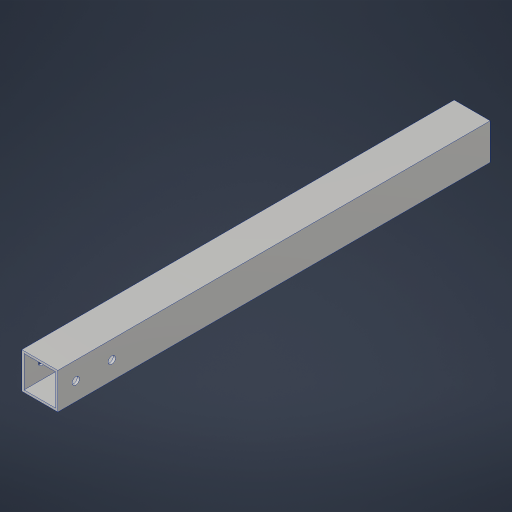
# Autodesk Inventor part: CL4-007
Saved by Autodesk Inventor 2023.4 (Build 274418000, 418)
## iProperties
RuleStatus: InUse
Created: 2025-02-03
Part Number: CL4-007
Material: Aluminum 6061
Document SubType Name: Modeling
Designer: brand
Mass: 304.185 g
Surface Area: 718.547 cm^2
Volume: 112.661 cm^3
Density: 2.7 g/cm^3
Appearance: Aluminum - Flat
AfterDocNew0: SHOW
AfterDocOpen0: SHOW
Author: brand
Autodesk Inventor part; units mm, degrees
ref_plane "YZ Plane" through (0, 0, 0) normal (1, 0, 0) x (0, 1, 0)
ref_plane "XZ Plane" through (0, 0, 0) normal (0, 1, 0) x (-1, 0, 0)
ref_plane "XY Plane" through (0, 0, 0) normal (0, 0, 1) x (1, 0, 0)
sketch "Sketch1" plane through (0, 0, 0) normal (0, 0, 1) x (1, 0, 0)
  line L0 (-12.7, -12.7) -> (12.7, -12.7)
  line L1 (12.7, -12.7) -> (12.7, 12.7)
  line L2 (12.7, 12.7) -> (-12.7, 12.7)
  line L3 (-12.7, 12.7) -> (-12.7, -12.7)
  line L4 (-12.7, -12.7) -> (12.7, 12.7) construction
  line L5 (12.7, -12.7) -> (-12.7, 12.7) construction
  line L6 (-11.1125, 11.1125) -> (11.1125, 11.1125)
  line L7 (11.1125, 11.1125) -> (11.1125, -11.1125)
  line L8 (11.1125, -11.1125) -> (-11.1125, -11.1125)
  line L9 (-11.1125, -11.1125) -> (-11.1125, 11.1125)
  point P0 (0, 0)
  dimension "width" = 25.4
  dimension "height" = 25.4
  dimension "thickness" = 1.5875
  constraints: 20 end point, 4 parallel, 2 midpoint, 2 perpendicular, 1 horizontal, 3 other
  measures "width" distance of L2.end L1.end
  measures "height" distance of L1.end L0.end
  measures "thickness" distance between parallel lines of L2 L6
extrude "Extrusion1" add sketch "Sketch1" along normal mid plane 304.8
sketch "Sketch2" plane through (12.7, -12.7, 152.4) normal (1, 0, 0) x (0, 0, -1)
  line L0 (304.8, 25.4) -> (304.8, 0) construction
  line L1 (304.8, 0) -> (0, 0) construction
  line L2 (0, 0) -> (0, 25.4) construction
  line L3 (0, 25.4) -> (304.8, 25.4) construction
  point P0 (152.4, 12.7)
  point P1 (12.7, 12.7)
  point P2 (38.1, 12.7)
  point P3 (0, 12.7)
  dimension "d5" = 25.4
  dimension "d6" = 12.7
  constraints: 2 horizontal alignment, 1 midpoint
  measures "d5" distance of point (38.1, 12.7) point (12.7, 12.7)
  measures "d6" distance from line of L2 point (12.7, 12.7)
hole "Hole1" at (12.7, 0, 139.7) at (12.7, 0, 114.3) direction (-1, 0, 0) diameter 5.1054 end through all clearance for "Flat Head Machine Screw (82)" size "#10" standard "Ansi Unified Screw Threads"
body "Solid1"
